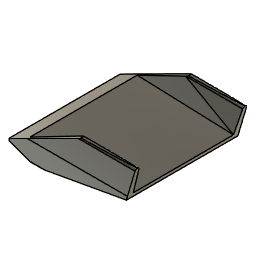
Downey-X-43A_stabilizer v7 (Autodesk Fusion 360 design; units mm, degrees)
Autodesk Fusion 360 part; units mm, degrees
sketch "Sketch7" plane through (0, 0, 0) normal (0, 1, 0) x (1, 0, 0)
  line L0 (2455.4576, -95.8693) -> (2455.4576, -76.2)
  line L1 (2455.4576, -76.2) -> (2651.76, 0)
  line L2 (2651.76, 0) -> (2706.624, 0)
  line L3 (2706.624, 0) -> (3456.432, -140.208)
  line L4 (3456.432, -140.208) -> (3535.68, -408.432)
  line L5 (3535.68, -408.432) -> (3066.288, -402.336)
  line L6 (3066.288, -402.336) -> (2455.4576, -95.8693)
  constraint vertical L0
  constraint horizontal L2
extrude "Extrude5" add sketch "Sketch7" along normal blind 950.976
sketch "Sketch8" plane through (0, 0, 0) normal (1, 0, 0) x (0, 1, 0)
  line L0 (950.976, 426.72) -> (0, 426.72)
  line L1 (475.488, 426.72) -> (475.488, -243.84)
  line L2 (1005.84, 457.2) -> (-54.0718, 457.2)
  line L3 (-54.0718, 457.2) -> (-54.0718, -231.5284)
  line L4 (-54.0718, -231.5284) -> (1005.84, -231.5284)
  line L5 (1005.84, -231.5284) -> (1005.84, 457.2)
  line L6 (911.352, 27.432) -> (933.2048, 2.8476)
  line L7 (938.5836, 2.5312) -> (943.1535, 6.5933)
  line L8 (944.4292, 9.2894) -> (950.976, 173.736)
  line L9 (950.976, 173.736) -> (950.976, 391.668)
  line L10 (917.448, 391.668) -> (902.208, 176.784)
  line L11 (902.208, 176.784) -> (475.488, 176.784)
  arc A0 (950.976, 391.668) -> (917.448, 391.668) centre (934.212, 391.668) ccw
  line L12 (911.352, 27.432) -> (475.488, 27.432)
  arc A1 (933.2048, 2.8476) -> (938.5836, 2.5312) centre (936.0524, 5.3789) ccw
  arc A2 (943.1535, 6.5933) -> (944.4292, 9.2894) centre (940.6223, 9.4409) ccw
  line L13 (48.768, 176.784) -> (475.488, 176.784)
  line L14 (33.528, 391.668) -> (48.768, 176.784)
  arc A3 (33.528, 391.668) -> (0, 391.668) centre (16.764, 391.668) ccw
  line L15 (0, 173.736) -> (0, 391.668)
  line L16 (6.5468, 9.2894) -> (0, 173.736)
  arc A4 (6.5468, 9.2894) -> (7.8225, 6.5933) centre (10.3537, 9.4409) ccw
  line L17 (12.3924, 2.5312) -> (7.8225, 6.5933)
  arc A5 (12.3924, 2.5312) -> (17.7712, 2.8476) centre (14.9236, 5.3789) ccw
  line L18 (39.624, 27.432) -> (17.7712, 2.8476)
  line L19 (39.624, 27.432) -> (475.488, 27.432)
  dimension "d19" = 3.81
  constraint midpoint L0 L1.start
  constraint perpendicular L0 L1
  constraint horizontal L2
  constraint vertical L3
  constraint horizontal L4
  constraint vertical L5
  constraint perpendicular L6 L7
  constraint vertical L9
  constraint tangent L9 A0
  constraint coincident L1 L11.end
  constraint perpendicular L1 L11
  constraint coincident L1 L12.end
  constraint perpendicular L1 L12
  constraint tangent L7 A1
  constraint tangent L6 A1
  constraint tangent L7 A2
  constraint tangent L8 A2
  constraint equal A1 A2
  constraint symmetric L9.end L1 A3.end
  constraint symmetric L1 L6.start L18.start
  constraint symmetric L1 L8.end L15.start
  constraint symmetric L1 L10.start L14.start
  constraint symmetric L1 L10.end L13.start
  constraint symmetric L1 L11.end L13.end
  constraint symmetric L1 A0 A3
  constraint symmetric L1 L12.end L19.end
  constraint symmetric L1 L7.start L17.start
  constraint symmetric L1 L6.end A5.end
  constraint symmetric L1 A1 A5
  constraint symmetric L1 L7.end A4.end
  constraint symmetric L1 L8.start L16.start
  constraint symmetric L1 A2 A4
  measures "d19" radius of A1
extrude "Extrude6" cut sketch "Sketch8" along normal blind 3962.4
ref_plane "WorkPlane3" through (3041.9851, 475.488, 481.584) normal (0, 0, 1) x (0, -1, 0)
sketch "Sketch10" plane through (0, 0, 481.584) normal (0, 0, 1) x (-1, 0, 0)
  line L0 (-2616.7317, -902.208) -> (-2616.7317, -48.768)
  line L1 (-2616.7317, -48.768) -> (-3467.2386, -48.768)
  line L2 (-3467.2386, -48.768) -> (-3467.2386, -902.208)
  line L3 (-3467.2386, -902.208) -> (-2616.7317, -902.208)
  line L4 (-2616.7317, -475.488) -> (-3627.1201, -475.488)
  line L5 (-2616.7317, -475.488) -> (-2616.7317, -932.688)
  line L6 (-2616.7317, -932.688) -> (-3467.2386, -902.208)
  line L7 (-3467.2386, -902.208) -> (-3467.2386, -475.488)
  line L8 (-2616.7317, -475.488) -> (-2616.7317, -18.288)
  line L9 (-2616.7317, -18.288) -> (-3467.2386, -48.768)
  line L10 (-3467.2386, -48.768) -> (-3467.2386, -475.488)
  constraint midpoint L0 L4.start
  constraint perpendicular L2 L4
  constraint perpendicular L3 L5
  constraint coincident L2.end L3.start
  constraint midpoint L2 L7.end
  constraint symmetric L5.start L4 L8.start
  constraint symmetric L4 L5.end L8.end
  constraint symmetric L4 L2.end L1.end
  constraint symmetric L4 L7.end L10.end
extrude "Extrude7" cut sketch "Sketch10" against normal blind 304.8 contours L3 L5 L6 | L1 L8 L9
